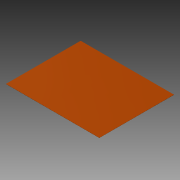
# Autodesk Inventor part: UltibotsKaptonHeater250x200
Saved by Autodesk Inventor 2015 SP1 (Build 190203100, 203)
## iProperties
Created: 2014-12-21
Part Number: UltibotsKaptonHeater250x200
Material: Generic
Document SubType Name: Modeling
Designer: Jack
Density: 1 g/cm^3
Appearance: Smooth - Light Orange
Mass: 26.84 g
Surface Area: 1009.42 cm^2
Volume: 26.84 cm^3
Catalog Web Link: http://www.ultibots.com/24v-kapton-heater-200mm-x-250mm/
Vendor: Ultibots
Author: Jack
Autodesk Inventor part; units mm, degrees
ref_plane "YZ Plane" through (0, 0, 0) normal (1, 0, 0) x (0, 1, 0)
ref_plane "XZ Plane" through (0, 0, 0) normal (0, 1, 0) x (-1, 0, 0)
ref_plane "XY Plane" through (0, 0, 0) normal (0, 0, 1) x (1, 0, 0)
sketch "Sketch1" plane through (0, 0, 0) normal (0, 0, 1) x (1, 0, 0)
  line L0 (0, 0) -> (250, 0)
  line L1 (250, 0) -> (250, 200)
  line L2 (250, 200) -> (0, 200)
  line L3 (0, 200) -> (0, 0)
  dimension "d0" = 250
  dimension "d1" = 200
  constraints: 8 end point, 2 parallel, 1 horizontal, 1 perpendicular
  measures "d0" distance of L2.end L1.end
  measures "d1" distance of L0.end L1.end
extrude "Extrusion1" add sketch "Sketch1" along normal blind 0.4
sketch "Sketch2" plane through (0, 0, 0) normal (0, 0, -1) x (-1, 0, 0)
  line L0 (0, 0) -> (-250, 0) projected
  line L1 (-250, 0) -> (-250, 200) projected
  line L2 (-96.5, 80) -> (-153.5, 80)
  line L3 (-153.5, 80) -> (-153.5, 120)
  line L4 (-153.5, 120) -> (-96.5, 120)
  line L5 (-96.5, 120) -> (-96.5, 80)
  dimension "d4" = 57
  dimension "d5" = 40
  dimension "d6" = 80
  dimension "d7" = 96.5
  constraints: 8 end point, 2 parallel, 1 horizontal, 1 perpendicular
  measures "d4" distance of L3.end L4.end
  measures "d5" distance of L2.end L3.end
  measures "d6" distance between parallel lines of L0 L2
  measures "d7" distance between parallel lines of L1 L3
extrude "Extrusion2" add sketch "Sketch2" along normal blind 3
body "Solid1"
